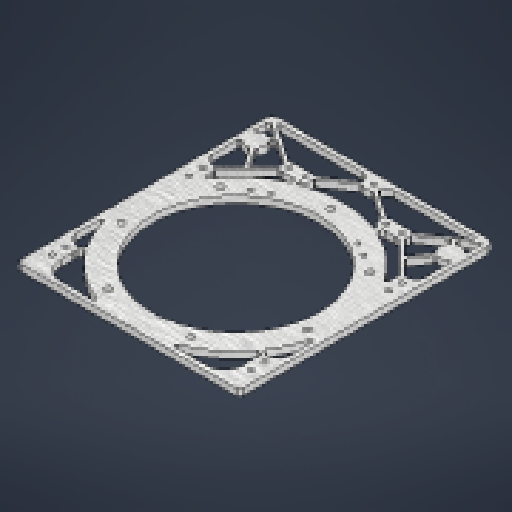
# Autodesk Inventor part: PLATE,SHOOTER,BOTTOM
Saved by Autodesk Inventor 2026 (Build 300175000, 175)
## iProperties
Created: 2026-01-27
Part Number: PLATE,SHOOTER,BOTTOM
Material: Aluminum 7075
Document SubType Name: Sheet Metal
Designer: Owen L
Density: 2.81 g/cm^3
Appearance: Satin - Brushed Heavy
Mass: 440.472 g
Surface Area: 731.077 cm^2
Volume: 156.751 cm^3
Sheet Metal Rule: Default
Author: Owen L
Autodesk Inventor part; units mm, degrees
ref_plane "YZ Plane" through (0, 0, 0) normal (1, 0, 0) x (0, 1, 0)
ref_plane "XZ Plane" through (0, 0, 0) normal (0, 1, 0) x (-1, 0, 0)
ref_plane "XY Plane" through (0, 0, 0) normal (0, 0, 1) x (1, 0, 0)
sketch "Sketch1" plane through (0, 0, 0) normal (0, 1, 0) x (-1, 0, 0)
  line L0 (-105.71734, 139.7) -> (105.71734, 139.7)
  line L1 (105.71734, 139.7) -> (105.71734, -139.7)
  line L2 (105.71734, -139.7) -> (-105.71734, -139.7)
  line L3 (-105.71734, -139.7) -> (-105.71734, 139.7)
  line L4 (-105.71734, 139.7) -> (105.71734, -139.7) construction
  line L5 (105.71734, 139.7) -> (-105.71734, -139.7) construction
  circle A0 centre (0, 37.794946) radius 79.375
  point P0 (0, 0)
  dimension "d0" = 211.43468
  dimension "d1" = 279.4
  dimension "d2" = 158.75
  dimension "d3" = 101.90505
  measures "d0" distance of L1.end L2.end
  measures "d1" distance of L0.end L1.end
  measures "d2" diameter of A0
  measures "d3" distance from line of L0 A0.centre
extrude "Plate1" add sketch "Sketch1" along normal blind 6.35
sketch "Sketch2" plane through (0, 0, 0) normal (0, -1, 0) x (1, 0, 0)
  point P0 (0, 0)
  point P1 (-41.275, -37.384203)
  point P2 (-38.4175, -66.594203)
  point P3 (-53.6575, -66.594203)
  point P4 (-53.6575, -30.399203)
  dimension "d7" = 37.3842
  dimension "d11" = 41.275
  dimension "d12" = 6.985
  dimension "d13" = 29.21
  dimension "d14" = 2.8575
  dimension "d15" = 12.3825
  constraints: 1 horizontal alignment, 1 vertical alignment
  measures "d7" vertical distance of point (-41.275, -37.384) point (0, 0)
  measures "d11" horizontal distance of point (0, 0) point (-41.275, -37.384)
  measures "d12" vertical distance of point (-53.658, -30.399) point (-41.275, -37.384)
  measures "d13" vertical distance of point (-38.418, -66.594) point (-41.275, -37.384)
  measures "d14" horizontal distance of point (-38.418, -66.594) point (-41.275, -37.384)
  measures "d15" horizontal distance of point (-53.658, -66.594) point (-41.275, -37.384)
hole "Hole1" at (-41.275, 0, -37.384203) at (-38.4175, 0, -66.594203) at (-53.6575, 0, -66.594203) at (-53.6575, 0, -30.399203) direction (0, 1, 0) diameter 4.2926 depth 6.35 clearance for "Flat Head Machine Screw" size "M4" standard "Ansi Metric M Profile"
mirror "Mirror1" about plane through (0, 0, 0) normal (1, 0, 0) of "Hole1"
sketch "Sketch3" plane through (0, 6.35, 0) normal (0, 1, 0) x (1, 0, 0)
  line L0 (105.71734, -139.7) -> (-105.71734, -139.7) construction
  line L1 (105.71734, 139.7) -> (105.71734, -139.7) construction
  line L2 (-105.71734, 139.7) -> (105.71734, 139.7) construction
  line L3 (0, -139.7) -> (0, 139.7) construction
  point P0 (0, 0)
  point P1 (94.60484, -117.475)
  point P2 (94.60484, -104.775)
  point P3 (94.60484, 12.7)
  point P4 (94.60484, 25.4)
  point P5 (-87.3125, 139.7)
  point P6 (-94.60484, -117.475)
  point P7 (-94.60484, -104.775)
  point P8 (-94.60484, 12.7)
  point P9 (-94.60484, 25.4)
  dimension "d23" = 22.225
  dimension "d24" = 12.7
  dimension "d25" = 11.1125
  dimension "d26" = 12.7
  dimension "d60" = 152.4
  constraints: 4 symmetric about line, 3 vertical alignment, 2 end point, 2 midpoint
  measures "d23" distance from line of L0 point (94.605, -117.475)
  measures "d24" distance of point (94.605, -104.775) point (94.605, -117.475)
  measures "d25" distance from line of L1 point (94.605, -117.475)
  measures "d26" distance of point (94.605, 25.4) point (94.605, 12.7)
  measures "d60" distance from line of L0 point (94.605, 12.7)
hole "Hole2" at (94.60484, 6.35, 117.475) at (94.60484, 6.35, 104.775) at (94.60484, 6.35, -12.7) at (94.60484, 6.35, -25.4) at (-94.60484, 6.35, -25.4) at (-94.60484, 6.35, -12.7) at (-94.60484, 6.35, 104.775) at (-94.60484, 6.35, 117.475) direction (0, -1, 0) diameter 4.9784 depth 6.35 clearance for "Flat Head Machine Screw (82)" size "#10" standard "Ansi Unified Screw Threads"
sketch "Sketch5" plane through (0, 6.35, 0) normal (0, 1, 0) x (1, 0, 0)
  line L0 (-105.71734, 139.7) -> (-105.71734, -139.7)
  line L1 (105.71734, 139.7) -> (105.71734, -139.7)
  line L2 (-105.71734, 139.7) -> (105.71734, 139.7)
  line L3 (105.71734, 139.7) -> (105.71734, 102.9208)
  line L4 (105.71734, 102.9208) -> (-105.71734, 102.9208)
  line L5 (-105.71734, 102.9208) -> (-105.71734, 139.7)
  point P0 (0, 0)
  dimension "d61" = 36.7792
  constraints: 8 end point, 2 parallel, 1 horizontal, 1 perpendicular, 1 point on line
  measures "d61" distance of L2.end L3.end
extrude "Cut2" cut sketch "Sketch5" against normal blind 6.35
fillet "Corner Round3" radius 6.35 2 edges at (-105.7173, 3.175, -102.9208) (105.7173, 3.175, -102.9208)
fillet "Corner Round3" radius 3.175 2 edges at (-105.7173, 3.175, 139.7) (105.7173, 3.175, 139.7)
sketch "Sketch6" plane through (0, 6.35, 0) normal (0, 1, 0) x (1, 0, 0)
  line L0 (99.36734, 102.9208) -> (-99.36734, 102.9208)
  point P0 (0, 0)
  point P1 (0, 93.3958)
  dimension "d66" = 9.525
  constraints: 1 vertical alignment
  measures "d66" distance from line of L0 point (0, 93.396)
hole "Hole3" at (0, 6.35, -93.3958) direction (0, -1, 0) diameter 4.9784 end through all clearance for "Flat Head Machine Screw (82)" size "#10" standard "Ansi Unified Screw Threads"
sketch "Sketch7" plane through (0, 6.35, 0) normal (0, 1, 0) x (1, 0, 0)
  circle A0 centre (0, 93.3958) radius 2.4892
  arc A1 (102.54234, -139.7) -> (105.71734, -136.525) centre (102.54234, -136.525) ccw
  line L0 (105.71734, 96.5708) -> (105.71734, -136.525)
  arc A2 (105.71734, 96.5708) -> (99.36734, 102.9208) centre (99.36734, 96.5708) ccw
  line L1 (99.36734, 102.9208) -> (-99.36734, 102.9208)
  arc A3 (-99.36734, 102.9208) -> (-105.71734, 96.5708) centre (-99.36734, 96.5708) ccw
  line L2 (-105.71734, -136.525) -> (-105.71734, 96.5708)
  arc A4 (-105.71734, -136.525) -> (-102.54234, -139.7) centre (-102.54234, -136.525) ccw
  line L3 (102.54234, -139.7) -> (-102.54234, -139.7)
  circle A5 centre (-94.60484, -117.475) radius 2.4892
  circle A6 centre (-94.60484, -104.775) radius 2.4892
  circle A7 centre (-94.60484, 12.7) radius 2.4892
  circle A8 centre (-94.60484, 25.4) radius 2.4892
  circle A9 centre (94.60484, 25.4) radius 2.4892
  circle A10 centre (94.60484, 12.7) radius 2.4892
  circle A11 centre (94.60484, -104.775) radius 2.4892
  circle A12 centre (94.60484, -117.475) radius 2.4892
  circle A13 centre (53.6575, 30.399203) radius 2.1463
  circle A14 centre (53.6575, 66.594203) radius 2.1463
  circle A15 centre (38.4175, 66.594203) radius 2.1463
  circle A16 centre (41.275, 37.384203) radius 2.1463
  circle A17 centre (-53.6575, 30.399203) radius 2.1463
  circle A18 centre (-53.6575, 66.594203) radius 2.1463
  circle A19 centre (-38.4175, 66.594203) radius 2.1463
  circle A20 centre (-41.275, 37.384203) radius 2.1463
  circle A21 centre (0, -37.794946) radius 79.375
  arc A22 (-99.36734, 98.1583) -> (-100.95484, 96.5708) centre (-99.36734, 96.5708) ccw
  line L4 (-99.36734, 98.1583) -> (99.36734, 98.1583)
  arc A23 (100.95484, 96.5708) -> (99.36734, 98.1583) centre (99.36734, 96.5708) ccw
  line L5 (100.95484, 96.5708) -> (100.95484, -134.9375)
  line L6 (100.95484, -134.9375) -> (-100.95484, -134.9375)
  line L7 (-100.95484, -134.9375) -> (-100.95484, 96.5708)
  circle A24 centre (0, -37.794946) radius 101.6
  circle A25 centre (94.60484, 12.7) radius 7.9375
  circle A26 centre (94.60484, 25.4) radius 7.9375
  circle A27 centre (-94.60484, 12.7) radius 7.9375
  circle A28 centre (-94.60484, 25.4) radius 7.9375
  circle A29 centre (-94.60484, -117.475) radius 7.9375
  circle A30 centre (-94.60484, -104.775) radius 7.9375
  circle A31 centre (94.60484, -117.475) radius 7.9375
  circle A32 centre (94.60484, -104.775) radius 7.9375
  circle A33 centre (53.6575, 66.594203) radius 6.35
  circle A34 centre (38.4175, 66.594203) radius 6.35
  circle A35 centre (0, 93.3958) radius 7.9375
  circle A36 centre (-38.4175, 66.594203) radius 6.35
  circle A37 centre (-53.6575, 66.594203) radius 2.1463
  circle A38 centre (-53.6575, 66.594203) radius 6.35
  line L8 (86.66734, -117.475) -> (86.66734, -104.775)
  line L9 (-86.66734, -117.475) -> (-86.66734, -104.775)
  line L10 (86.66734, 25.4) -> (86.66734, 12.7)
  line L11 (53.6575, 60.244203) -> (38.4175, 60.244203)
  line L12 (38.4175, 72.944203) -> (53.6575, 72.944203)
  line L13 (-38.4175, 72.944203) -> (-53.6575, 72.944203)
  line L14 (-53.6575, 60.244203) -> (-38.4175, 60.244203)
  line L15 (-86.66734, 12.7) -> (-86.66734, 25.4)
  arc A39 (-86.66734, -117.475) -> (-69.20484, -134.9375) centre (-69.20484, -117.475) ccw
  arc A40 (69.20484, -134.9375) -> (86.66734, -117.475) centre (69.20484, -117.475) ccw
  arc A41 (93.81109, 33.297713) -> (86.66734, 25.4) centre (94.60484, 25.4) ccw
  arc A42 (93.81109, 33.297713) -> (100.95484, 41.195426) centre (93.01734, 41.195426) ccw
  arc A43 (-86.66734, 25.4) -> (-93.81109, 33.297713) centre (-94.60484, 25.4) ccw
  arc A44 (-100.95484, 41.195426) -> (-93.81109, 33.297713) centre (-93.01734, 41.195426) ccw
  line L16 (0, 85.4583) -> (-7.653832, 85.4583) construction
  line L17 (0, 85.4583) -> (6.78815, 85.4583) construction
  arc A45 (-7.77713, 91.8083) -> (0, 85.4583) centre (0, 93.3958) ccw
  arc A46 (-7.77713, 91.8083) -> (-15.55426, 98.1583) centre (-15.55426, 90.2208) ccw
  arc A47 (0, 85.4583) -> (7.77713, 91.8083) centre (0, 93.3958) ccw
  arc A48 (15.55426, 98.1583) -> (7.77713, 91.8083) centre (15.55426, 90.2208) ccw
  arc A49 (-86.66734, -104.775) -> (-93.81109, -96.877287) centre (-94.60484, -104.775) ccw
  arc A50 (-100.95484, -88.979574) -> (-93.81109, -96.877287) centre (-93.01734, -88.979574) ccw
  arc A51 (93.81109, -96.877287) -> (86.66734, -104.775) centre (94.60484, -104.775) ccw
  arc A52 (93.81109, -96.877287) -> (100.95484, -88.979574) centre (93.01734, -88.979574) ccw
  arc A53 (1.424228, 91.354307) -> (-1.424228, 95.437293) centre (0, 93.3958) ccw
  line L18 (-53.6575, 66.594203) -> (-94.60484, 25.4) construction
  line L19 (-54.783401, 67.713356) -> (-95.730741, 26.519153)
  line L20 (-93.478939, 24.280847) -> (-52.531599, 65.475049)
  arc A54 (-52.531599, 65.475049) -> (-54.783401, 67.713356) centre (-53.6575, 66.594203) ccw
  arc A55 (-95.730741, 26.519153) -> (-93.478939, 24.280847) centre (-94.60484, 25.4) ccw
  line L21 (-53.6575, 66.594203) -> (-104.476969, 100.340972) construction
  line L22 (-52.779309, 67.916676) -> (-103.598778, 101.663445)
  line L23 (-105.35516, 99.018498) -> (-54.535691, 65.271729)
  arc A56 (-54.535691, 65.271729) -> (-52.779309, 67.916676) centre (-53.6575, 66.594203) ccw
  arc A57 (-103.598778, 101.663445) -> (-105.35516, 99.018498) centre (-104.476969, 100.340972) ccw
  line L24 (-38.4175, 66.594203) -> (-41.275, 37.384203) construction
  line L25 (-39.997458, 66.748764) -> (-42.854958, 37.538764)
  line L26 (-39.695042, 37.229642) -> (-36.837542, 66.439642)
  arc A58 (-36.837542, 66.439642) -> (-39.997458, 66.748764) centre (-38.4175, 66.594203) ccw
  arc A59 (-42.854958, 37.538764) -> (-39.695042, 37.229642) centre (-41.275, 37.384203) ccw
  line L27 (38.4175, 66.594203) -> (41.275, 37.384203) construction
  line L28 (36.281397, 66.385236) -> (39.138897, 37.175236)
  line L29 (43.411103, 37.593169) -> (40.553603, 66.803169)
  arc A60 (40.553603, 66.803169) -> (36.281397, 66.385236) centre (38.4175, 66.594203) ccw
  arc A61 (39.138897, 37.175236) -> (43.411103, 37.593169) centre (41.275, 37.384203) ccw
  line L30 (38.4175, 66.594203) -> (0, 93.3958) construction
  line L31 (39.325808, 67.896175) -> (0.908308, 94.697772)
  line L32 (-0.908308, 92.093828) -> (37.509192, 65.29223)
  arc A62 (37.509192, 65.29223) -> (39.325808, 67.896175) centre (38.4175, 66.594203) ccw
  arc A63 (0.908308, 94.697772) -> (-0.908308, 92.093828) centre (0, 93.3958) ccw
  line L33 (53.6575, 66.594203) -> (94.60484, 25.4) construction
  line L34 (52.531599, 65.475049) -> (93.478939, 24.280847)
  line L35 (95.730741, 26.519153) -> (54.783401, 67.713356)
  arc A64 (54.783401, 67.713356) -> (52.531599, 65.475049) centre (53.6575, 66.594203) ccw
  arc A65 (93.478939, 24.280847) -> (95.730741, 26.519153) centre (94.60484, 25.4) ccw
  line L36 (53.6575, 66.594203) -> (103.857468, 101.060928) construction
  line L37 (54.556054, 65.28548) -> (104.756022, 99.752205)
  line L38 (102.958914, 102.369651) -> (52.758946, 67.902926)
  arc A66 (52.758946, 67.902926) -> (54.556054, 65.28548) centre (53.6575, 66.594203) ccw
  arc A67 (104.756022, 99.752205) -> (102.958914, 102.369651) centre (103.857468, 101.060928) ccw
  line L39 (-38.4175, 66.594203) -> (0, 93.3958) construction
  line L40 (-37.509192, 65.29223) -> (0.908308, 92.093828)
  line L41 (-0.908308, 94.697772) -> (-39.325808, 67.896175)
  arc A68 (-39.325808, 67.896175) -> (-37.509192, 65.29223) centre (-38.4175, 66.594203) ccw
  arc A69 (0.908308, 92.093828) -> (-0.908308, 94.697772) centre (0, 93.3958) ccw
  line L42 (-94.60484, -104.775) -> (0, -37.794946) construction
  line L43 (-93.687527, -106.070644) -> (0.917313, -39.09059)
  line L44 (-0.917313, -36.499302) -> (-95.522153, -103.479356)
  arc A70 (-95.522153, -103.479356) -> (-93.687527, -106.070644) centre (-94.60484, -104.775) ccw
  arc A71 (0.917313, -39.09059) -> (-0.917313, -36.499302) centre (0, -37.794946) ccw
  line L45 (94.60484, -104.775) -> (0, -37.794946) construction
  line L46 (95.522153, -103.479356) -> (0.917313, -36.499302)
  line L47 (-0.917313, -39.09059) -> (93.687527, -106.070644)
  arc A72 (93.687527, -106.070644) -> (95.522153, -103.479356) centre (94.60484, -104.775) ccw
  arc A73 (0.917313, -36.499302) -> (-0.917313, -39.09059) centre (0, -37.794946) ccw
  circle A74 centre (-92.25534, 73.7108) radius 9.525
  line L48 (-92.25534, 73.7108) -> (-83.723206, 86.559394) construction
  line L49 (-90.932866, 72.832609) -> (-82.400732, 85.681203)
  line L50 (-85.045679, 87.437585) -> (-93.577814, 74.588991)
  arc A75 (-93.577814, 74.588991) -> (-90.932866, 72.832609) centre (-92.25534, 73.7108) ccw
  arc A76 (-82.400732, 85.681203) -> (-85.045679, 87.437585) centre (-83.723206, 86.559394) ccw
  line L51 (-92.25534, 73.7108) -> (-74.13117, 45.997101) construction
  line L52 (-93.583949, 72.841918) -> (-75.459779, 45.12822)
  line L53 (-72.802561, 46.865983) -> (-90.926731, 74.579682)
  arc A77 (-90.926731, 74.579682) -> (-93.583949, 72.841918) centre (-92.25534, 73.7108) ccw
  arc A78 (-75.459779, 45.12822) -> (-72.802561, 46.865983) centre (-74.13117, 45.997101) ccw
  line L54 (0, 102.9208) -> (0, -139.7) construction
  circle A79 centre (92.25534, 73.7108) radius 9.525
  line L55 (90.932866, 72.832609) -> (82.400732, 85.681203)
  line L56 (85.045679, 87.437585) -> (93.577814, 74.588991)
  line L57 (92.25534, 73.7108) -> (74.13117, 45.997101) construction
  line L58 (93.583949, 72.841918) -> (75.459779, 45.12822)
  line L59 (72.802561, 46.865983) -> (90.926731, 74.579682)
  point P0 (0, 0)
  point P1 (-74.13117, 45.997101)
  point P2 (-79.067234, 83.467587)
  point P3 (-100.489872, 97.693332)
  point P4 (-39.84625, 51.989203)
  point P5 (39.84625, 51.989203)
  point P6 (19.20875, 79.995001)
  point P7 (74.13117, 45.997101)
  point P8 (78.757484, 83.827565)
  point P9 (-19.20875, 79.995001)
  point P10 (-47.30242, -71.284973)
  point P11 (47.30242, -71.284973)
  point P12 (83.828384, -95.200189)
  point P13 (89.174822, -98.985457)
  point P14 (100.95484, -49.226494)
  point P15 (87.340195, -101.576744)
  point P16 (81.993758, -97.791477)
  point P17 (29.763807, -134.9375)
  point P18 (100.869646, 97.083863)
  point P19 (59.624717, 68.765566)
  point P20 (59.117863, 63.352762)
  point P21 (90.248031, 32.034917)
  point P22 (93.81109, 33.297713)
  point P23 (87.99623, 29.79661)
  point P24 (56.866062, 61.114456)
  point P25 (41.195241, 60.244203)
  point P26 (41.723669, 54.842495)
  point P27 (86.66734, 15.227051)
  point P28 (57.827609, 71.383012)
  point P29 (96.82518, 98.1583)
  point P30 (7.77713, 91.8083)
  point P31 (7.286644, 90.247988)
  point P32 (34.283291, 71.414039)
  point P33 (-5.470028, 87.644043)
  point P34 (-32.466674, 68.810094)
  point P35 (-37.436155, 60.320491)
  point P36 (-37.809124, 56.507918)
  point P37 (37.224949, 56.740038)
  point P38 (36.863255, 60.437351)
  point P39 (32.466674, 68.810094)
  point P40 (5.470028, 87.644043)
  point P41 (-34.283291, 71.414039)
  point P42 (-7.286644, 90.247988)
  point P43 (-7.77713, 91.8083)
  point P44 (-98.320358, 98.1583)
  point P45 (-57.901227, 71.317896)
  point P46 (-59.657609, 68.672949)
  point P47 (-100.95484, 96.096457)
  point P48 (-93.81109, 33.297713)
  point P49 (-90.248031, 32.034917)
  point P50 (-59.117863, 63.352762)
  point P51 (-41.136551, 55.1047)
  point P52 (-40.633774, 60.244203)
  point P53 (-56.866062, 61.114456)
  point P54 (-87.99623, 29.79661)
  point P55 (-86.66734, 15.227051)
  point P56 (-89.174822, -98.985457)
  point P57 (-83.828384, -95.200189)
  point P58 (-100.95484, -49.226494)
  point P59 (-29.763807, -134.9375)
  point P60 (-81.993758, -97.791477)
  point P61 (-87.340195, -101.576744)
  point P62 (-87.989273, 80.135097)
  point P63 (-83.193255, 59.853951)
  point P64 (-76.163531, 46.204329)
  point P65 (-88.443575, 64.981764)
  point P66 (-100.95484, 69.832099)
  point P67 (-88.382364, 82.412851)
  point P68 (-85.923871, 86.115112)
  point P69 (-85.786358, 66.719528)
  point P70 (-73.875318, 48.506337)
  point P71 (-83.278923, 84.358729)
  point P72 (-85.737417, 80.656468)
  point P73 (85.786358, 66.719528)
  point P74 (85.737417, 80.656468)
  point P75 (82.983577, 84.803493)
  point P76 (73.875318, 48.506337)
  point P77 (100.95484, 69.832099)
  point P78 (88.443575, 64.981764)
  point P79 (76.163531, 46.204329)
  point P80 (85.601337, 86.600817)
  point P81 (88.382364, 82.412851)
  point P82 (-82.845014, 87.881868)
  point P83 (-100.95484, 77.589501)
  point P84 (100.95484, 77.589501)
  dimension "d75" = 15.875
  dimension "d74" = 4.7625
  dimension "d76" = 12.7
  dimension "d77" = 7.9375
  dimension "d78" = 4.9784
  dimension "d79" = 3.175
  dimension "d80" = 3.175
  dimension "d81" = 3.175
  dimension "d82" = 4.2926
  dimension "d83" = 3.175
  dimension "d84" = 3.175
  dimension "d85" = 3.175
  dimension "d86" = 3.175
  dimension "d87" = 3.175
  dimension "d88" = 3.175
  dimension "d92" = 13.462
  dimension "d93" = 29.21
  dimension "d94" = 3.175
  dimension "d95" = 3.175
  dimension "d96" = 19.05
  dimension "d97" = 19.05
  dimension "d103" = 203.2
  constraints: 138 end point, 93 point on circle, 67 tangent, 48 centre point, 23 equal radius, 16 point on line, 15 midpoint, 14 coincident, 12 parallel, 10 symmetric about line, 5 vertical, 4 horizontal, 4 horizontal alignment, 1 perpendicular, 28 other
  measures "d74" distance between parallel lines of L2 L7
  measures "d76" diameter of A33
  measures "d77" radius of A42
  measures "d78" diameter of A53
  measures "d79" diameter of A55
  measures "d80" diameter of A57
  measures "d81" diameter of A59
  measures "d82" diameter of A61
  measures "d83" diameter of A63
  measures "d84" diameter of A65
  measures "d85" diameter of A67
  measures "d86" diameter of A69
  measures "d87" diameter of A71
  measures "d88" diameter of A73
  measures "d92" distance from line of L2 L48.start
  measures "d93" distance from line of L1 L48.start
  measures "d94" diameter of A76
  measures "d95" diameter of A78
  measures "d96" diameter of A74
  measures "d97" diameter of A79
  measures "d103" diameter of A24
extrude "Cut3" cut sketch "Sketch7" against normal blind 6.35 contours L32 A34 L28 A24 L26 A36 L40 A35 | A35 A48 L4 L38 A33 L12 A34 L31 | L41 A36 L13 A38 L22 L4 A46 A35 | L11 A33 L34 A26 L10 A24 L29 | A24 L15 A28 L20 A38 L14 L25 | A23 L5 A79 L56 L37 | L37 L55 A79 L59 L35 A33 | A38 L19 L53 A74 L49 L23 | L35 L58 A79 L5 A42 A26 | L23 L50 A74 L7 | L5 A52 A32 L46 A24 | A28 A44 L7 A74 L52 L19 | A24 L44 A30 A50 L7 | L47 A32 L8 A40 L6 A24 | A24 L6 A39 L9 A30 L43
fillet "Corner Round4" radius 1.5875 66 edges at (-100.9548, 3.175, 49.2265) (-89.1748, 3.175, 98.9855) (-83.8284, 3.175, 95.2002) (-81.9938, 3.175, 97.7915) (-87.3402, 3.175, 101.5767) (-29.7638, 3.175, 134.9375) (87.3402, 3.175, 101.5767) (89.1748, 3.175, 98.9855) (81.9938, 3.175, 97.7915) (29.7638, 3.175, 134.9375) (83.8284, 3.175, 95.2002) (100.9548, 3.175, 49.2265) (87.9962, 3.175, -29.7966) (90.248, 3.175, -32.0349) (56.8661, 3.175, -61.1145) (59.1179, 3.175, -63.3528) (32.4667, 3.175, -68.8101) (36.8633, 3.175, -60.4374) (37.2249, 3.175, -56.74) (41.7237, 3.175, -54.8425) (-87.9962, 3.175, -29.7966) (-32.4667, 3.175, -68.8101) (-5.47, 3.175, -87.644) (5.47, 3.175, -87.644) (-41.1366, 3.175, -55.1047) (-86.6673, 3.175, -15.2271) (7.2866, 3.175, -90.248) (34.2833, 3.175, -71.414) (41.1952, 3.175, -60.2442) (57.8276, 3.175, -71.383) (-98.3204, 3.175, -98.1583) (-34.2833, 3.175, -71.414) (-7.2866, 3.175, -90.248) (59.6247, 3.175, -68.7656) (100.8696, 3.175, -97.0839) (96.8252, 3.175, -98.1583) (86.6673, 3.175, -15.2271) (-59.6576, 3.175, -68.6729) (-100.9548, 3.175, -96.0965) (-57.9012, 3.175, -71.3179) (-37.4362, 3.175, -60.3205) (-37.8091, 3.175, -56.5079) (-40.6338, 3.175, -60.2442) (-59.1179, 3.175, -63.3528) (-90.248, 3.175, -32.0349) (-56.8661, 3.175, -61.1145) (-100.9548, 3.175, -69.8321) (-88.4436, 3.175, -64.9818) (-76.1635, 3.175, -46.2043) (-85.7864, 3.175, -66.7195) (-85.7374, 3.175, -80.6565) (-83.2789, 3.175, -84.3587) (-73.8753, 3.175, -48.5063) (-88.3824, 3.175, -82.4129) (-85.9239, 3.175, -86.1151) (-100.9548, 3.175, -77.5895) (85.7374, 3.175, -80.6565) (85.7864, 3.175, -66.7195) (73.8753, 3.175, -48.5063) (82.9836, 3.175, -84.8035) (76.1635, 3.175, -46.2043) (88.4436, 3.175, -64.9818) (100.9548, 3.175, -69.8321) (88.3824, 3.175, -82.4129) (85.6013, 3.175, -86.6008) (100.9548, 3.175, -77.5895)
sketch "Sketch8" plane through (0, 0, 0) normal (0, -1, 0) x (1, 0, 0)
  circle A0 centre (0, 37.794946) radius 79.375
  point P0 (0, 0)
  point P1 (0, -52.692554)
  point P2 (70.745976, -18.623087)
  point P3 (88.218789, 57.930309)
  point P4 (39.261055, 119.321366)
  point P5 (-39.261055, 119.321366)
  point P6 (-88.218789, 57.930309)
  point P7 (-70.745976, -18.623087)
  dimension "d100" = 360
  dimension "d102" = 90.4875
  constraints: 1 vertical alignment, 8 other
  measures "d102" distance of A0.centre point (0, -52.693)
hole "Hole4" at (0, 0, -52.692554) at (70.745976, 0, -18.623087) at (88.218789, 0, 57.930309) at (39.261055, 0, 119.321366) at (-39.261055, 0, 119.321366) at (-88.218789, 0, 57.930309) at (-70.745976, 0, -18.623087) direction (0, 1, 0) diameter 6.35 end through all
equation "\"d21\" = Thickness"
equation "\"d34\" = Thickness"
equation "\"d4\" = Thickness"
equation "\"BendRadius\" = Thickness"
equation "\"BendReliefWidth\" = Thickness"
equation "\"BendReliefDepth\" = 0.5 * Thickness"
equation "\"CornerReliefSize\" = 4 * Thickness"
equation "\"MinimumRemnant\" = 2 * Thickness"
equation "\"TransitionRadius\" = BendRadius"
equation "\"JacobiRadiusSize\" = BendRadius"
equation "\"GapSize\" = Thickness"
equation "\"Thickness\" = 6.35"
body "Solid1"
